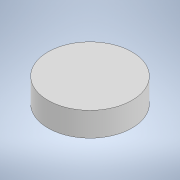
# Autodesk Inventor part: тест
Saved by Autodesk Inventor 2022 (Build 260153070, 153G)
## iProperties
Created: 2021-09-16
Part Number: тест
Material: Типовые
Document SubType Name: Modeling
Designer: Алексанян Г.
Density: 1 g/cm^3
Appearance: По умолчанию
Author: Алексанян Г.
Autodesk Inventor part; units mm, degrees
ref_plane "YZ Plane" through (0, 0, 0) normal (1, 0, 0) x (0, 1, 0)
ref_plane "XZ Plane" through (0, 0, 0) normal (0, 1, 0) x (-1, 0, 0)
ref_plane "XY Plane" through (0, 0, 0) normal (0, 0, 1) x (1, 0, 0)
sketch "Эскиз1" plane through (0, 0, 0) normal (0, 1, 0) x (-1, 0, 0)
  circle A0 centre (6.6012, 5.1547) radius 17.4408
  point P0 (0, 0)
  dimension "d0" = 10
  constraints: 1 centre point
extrude "Выдавливание1" add sketch "Эскиз1" along normal blind 10
